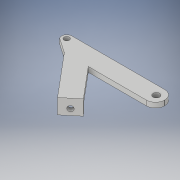
# Autodesk Inventor part: ventilador controladora_suportV
Saved by Autodesk Inventor 2019 (Build 230136000, 136)
## iProperties
Created: 2018-08-15
Part Number: ventilador controladora_suportV
Material: Genérico
Document SubType Name: Modeling
Designer: Albert Garangou Culebras
Density: 1 g/cm^3
Appearance: Valor por defecto
Author: Albert Garangou Culebras
Autodesk Inventor part; units mm, degrees
ref_plane "YZ Plane" through (0, 0, 0) normal (1, 0, 0) x (0, 1, 0)
ref_plane "XZ Plane" through (0, 0, 0) normal (0, 1, 0) x (-1, 0, 0)
ref_plane "XY Plane" through (0, 0, 0) normal (0, 0, 1) x (1, 0, 0)
sketch "Boceto1" plane through (0, 0, 0) normal (0, 1, 0) x (-1, 0, 0)
  line L0 (-2.031, 0) -> (-63, 0)
  line L1 (-65, -2) -> (-65, -8.0305)
  line L2 (-62.8998, -10.9676) -> (-2.0305, -10.9676)
  line L3 (0, -8.9987) -> (0, -2.031)
  line L4 (0, -8.9987) -> (0, -10.9676)
  line L5 (0, -10.9676) -> (-2.0305, -10.9676)
  line L6 (0, -2.031) -> (0, 0)
  line L7 (-65, -8.0305) -> (-65, -10.9676)
  line L8 (-65, -10.9676) -> (-62.8998, -10.9676)
  line L9 (-65, -2) -> (-65, 0)
  line L10 (-63, 0) -> (-65, 0)
  line L11 (0, 0) -> (-2.031, 0)
  dimension "d0" = 65
  constraints: 24 end point, 4 perpendicular, 4 point on line, 4 vertical, 3 horizontal
  measures "d0" distance of L6.end L9.end
extrude "Extrusión1" add sketch "Boceto1" along normal blind 3
sketch "Boceto2" plane through (0, 3, 0) normal (0, 1, 0) x (1, 0, 0)
  line L0 (0, 10.9676) -> (0, 0) projected
  circle A0 centre (5, 5.4838) radius 2
  line L1 (65, 0) -> (65, 10.9676) projected
  circle A1 centre (60, 5.4838) radius 2
  line L2 (65, 5.4838) -> (60, 5.4838)
  line L3 (0, 5.4838) -> (5, 5.4838)
  point P0 (0.1384, 8.9976)
  point P1 (0.0312, 2.0308)
  point P2 (65, 2)
  point P3 (65, 8.0305)
  dimension "d20" = 5
  dimension "d31" = 4
  dimension "d32" = 4
  constraints: 4 end point, 2 centre point, 2 horizontal, 1 coincident, 1 midpoint, 2 other
  measures "d20" distance of L2.start L2.end
  measures "d31" diameter of A0
  measures "d32" diameter of A1
extrude "Extrusión2" cut sketch "Boceto2" against normal blind 5
sketch "Boceto3" plane through (0, 3, 0) normal (0, 1, 0) x (1, 0, 0)
  circle A0 centre (5, 5.4838) radius 2 projected
  line L0 (5, 5.4838) -> (319.2562, 5.4838) construction
  line L1 (19.8683, -0.0721) -> (38.3706, -22.1223)
  line L2 (16.8683, -0.0721) -> (16.8078, 0)
  line L3 (11.4418, -7.1428) -> (5.4483, 0)
  line L4 (65, 0) -> (0, 0) projected
  line L5 (11.4418, -7.1428) -> (29.9441, -29.1929)
  line L6 (38.3706, -22.1223) -> (29.9441, -29.1929)
  line L7 (16.8078, 0) -> (19.8078, 0)
  line L8 (0, 0) -> (65, 0) projected
  dimension "d37" = 3
  constraints: 14 end point, 1 horizontal, 1 perpendicular, 1 point on line
  measures "d37" distance of L2.end L7.end
extrude "Extrusión3" add sketch "Boceto3" against normal blind 3
sketch "Boceto10" plane through (0, 3, 0) normal (0, 1, 0) x (1, 0, 0)
  line L0 (6.3645, 0) -> (-0.0991, 7.9201)
  line L1 (-0.0991, 7.9201) -> (0, 3)
  line L2 (2.4483, 0) -> (6.3645, 0)
  line L3 (65, 0) -> (0, 0) projected
  line L4 (2.4483, 0) -> (0, 0)
  line L5 (0, 0) -> (0, 3)
  constraints: 10 end point, 1 collinear, 1 perpendicular
extrude "Extrusión9" cut sketch "Boceto10" against normal blind 39
fillet "Empalme8" radius 5.48 2 edges at (65, 1.5, 0) (65, 1.5, -10.9676)
fillet "Empalme10" radius 3 2 edges at (0, 1.5, -7.7987) (0, 1.5, -10.9676)
sketch "Boceto11" plane through (0, 3, 0) normal (0, 1, 0) x (1, 0, 0)
  line L0 (0, 0) -> (0, 10.9676) projected
  line L1 (0, 3) -> (0, 0)
  line L2 (0, 0) -> (2.4483, 0)
  line L3 (2.4483, 0) -> (0, 3) projected
  line L4 (2.4483, 0) -> (0, 3)
  constraints: 6 end point, 2 collinear, 1 perpendicular
extrude "Extrusión10" cut sketch "Boceto11" against normal blind 57.75
sketch "Boceto13" plane through (0, 3, 0) normal (0, 1, 0) x (1, 0, 0)
  arc A0 (3.7344, 10.9676) -> (1.4102, 6.0708) centre (3.7344, 7.9676) ccw projected
  circle A1 centre (3.7344, 7.9676) radius 1.6
  point P0 (0, 0)
  dimension "d55" = 3.2
  constraints: 1 centre point, 1 coincident
  measures "d55" diameter of A1
extrude "Extrusión12" cut sketch "Boceto13" against normal blind 8
sketch "Boceto14" plane through (0, 3, 0) normal (0, 1, 0) x (1, 0, 0)
  line L0 (34.4548, -16.3636) -> (37.6687, -20.1938) projected
  line L1 (37.6687, -20.1938) -> (35.7403, -17.8957)
  line L2 (37.6687, -20.1938) -> (39.9668, -18.2655)
  line L3 (39.9668, -18.2655) -> (24.6403, 0)
  line L4 (39.9668, -18.2655) -> (31.5403, -25.3361)
  line L5 (29.2422, -27.2645) -> (37.6687, -20.1938) projected
  line L6 (31.5403, -25.3361) -> (10.2808, 0)
  line L7 (10.2808, 0) -> (24.6403, 0)
  point P0 (0, 0)
  dimension "d58" = 3
  dimension "d59" = 3
  dimension "d60" = 11
  constraints: 12 end point, 2 point on line, 1 horizontal, 1 perpendicular
  measures "d58" distance of L0.end L1.end
  measures "d59" distance of L0.end L2.end
  measures "d60" distance of L2.end L4.end
extrude "Extrusión13" add sketch "Boceto14" against normal blind 3
sketch "Boceto15" plane through (0, 0, 0) normal (0, -1, 0) x (1, 0, 0)
  line L0 (31.5403, 25.3361) -> (10.2808, 0) projected
  line L1 (31.5403, 25.3361) -> (29.612, 23.038)
  line L2 (29.612, 23.038) -> (38.0385, 15.9673)
  line L3 (24.6403, 0) -> (39.9668, 18.2655) projected
  line L4 (39.9668, 18.2655) -> (31.5403, 25.3361)
  line L5 (31.5403, 25.3361) -> (39.9668, 18.2655) projected
  point P0 (0, 0)
  dimension "d63" = 3
  constraints: 6 end point, 4 point on line, 1 perpendicular
  measures "d63" distance of L0.start L1.end
extrude "Extrusión14" add sketch "Boceto15" along normal blind 6
sketch "Boceto16" plane through (31.5403, -6, 25.3361) normal (0.6427876, 0, 0.7660444) x (0.7660444, 0, -0.6427876)
  line L0 (0, 9) -> (11, 9) projected
  line L1 (5.5, 9) -> (5.5, 0)
  line L2 (2.035, 6) -> (44.7692, 6) projected
  line L3 (5.5, 6) -> (5.5, 5.2)
  line L4 (5.5, 5.2) -> (5.5, 2)
  line L5 (5.5, 2) -> (5.5, 0)
  circle A0 centre (5.5, 3.6) radius 1.6
  point P0 (-7.8755, 6)
  dimension "d66" = 0.8
  dimension "d67" = 3.2
  constraints: 8 end point, 4 point on line, 2 midpoint, 1 collinear, 1 vertical, 1 vertical alignment, 2 other
  measures "d66" distance of L3.start L3.end
  measures "d67" distance of L3.end L4.end
extrude "Extrusión15" cut sketch "Boceto16" against normal blind 26.05
sketch "Boceto17" plane through (0, 3, 0) normal (0, 1, 0) x (1, 0, 0)
  line L0 (1.4102, 6.0708) -> (6.3645, 0) projected
  line L1 (10.2892, 0) -> (1.4102, 6.0708)
  line L2 (1.4102, 6.0708) -> (6.3645, 0)
  line L3 (6.3645, 0) -> (10.2892, 0)
  point P0 (0, 0)
  constraints: 6 end point, 1 collinear, 1 horizontal
extrude "Extrusión16" cut sketch "Boceto17" against normal blind 59.45
